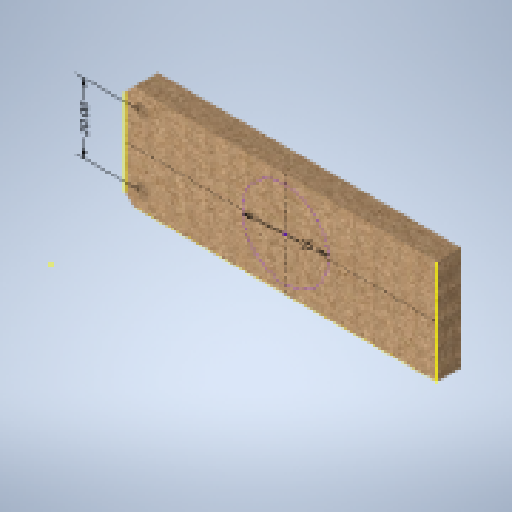
# Autodesk Inventor part: Dedo
Saved by Autodesk Inventor 2023.1 (Build 271208000, 208)
## iProperties
Created: 2022-10-28
Part Number: Dedo
Material: MDF Medium Density Fiberboard
Document SubType Name: Modeling
Designer: Daniel Peña
Density: 0.8 g/cm^3
Appearance: Cardboard - Corrugated
Author: Daniel Peña
Autodesk Inventor part; units mm, degrees
ref_plane "YZ Plane" through (0, 0, 0) normal (1, 0, 0) x (0, 1, 0)
ref_plane "XZ Plane" through (0, 0, 0) normal (0, 1, 0) x (-1, 0, 0)
ref_plane "XY Plane" through (0, 0, 0) normal (0, 0, 1) x (1, 0, 0)
sketch "Sketch1" plane through (0, 0, 0) normal (0, 0, 1) x (1, 0, 0)
  line L0 (23.8989, 56.2562) -> (111.3989, 56.2562)
  line L1 (111.3989, 56.2562) -> (111.3989, 26.2562)
  line L2 (111.3989, 26.2562) -> (23.8989, 26.2562)
  line L3 (21.3989, 28.7562) -> (21.3989, 53.7562)
  line L4 (21.3989, 53.7562) -> (23.8989, 56.2562)
  line L5 (21.3989, 28.7562) -> (23.8989, 26.2562)
  point P0 (0, 0)
  point P1 (21.3989, 56.2562)
  point P2 (21.3989, 26.2562)
  dimension "d0" = 30
  dimension "d1" = 90
  dimension "d2" = 2.5
  dimension "d3" = 2.5
  dimension "d4" = 2.5
  dimension "d5" = 2.5
  constraints: 12 end point, 4 point on line, 2 parallel, 1 horizontal, 1 perpendicular
  measures "d0" distance of L0.end L1.end
  measures "d1" distance of L1.end point (21.399, 26.256)
  measures "d2" distance of L3.end point (21.399, 56.256)
  measures "d3" distance of L0.start point (21.399, 56.256)
  measures "d4" distance of L3.start point (21.399, 26.256)
  measures "d5" distance of L2.end point (21.399, 26.256)
extrude "Extrusion1" add sketch "Sketch1" along normal blind 7
sketch "Sketch2" plane through (0, 0, 7) normal (0, 0, 1) x (1, 0, 0)
  line L0 (111.3989, 26.2562) -> (111.3989, 56.2562) construction
  line L1 (111.3989, 41.2562) -> (21.3989, 41.2562) construction
  line L2 (21.3989, 53.7562) -> (21.3989, 28.7562) construction
  line L3 (23.8989, 26.2562) -> (111.3989, 26.2562) projected
  point P0 (0, 0)
  point P1 (26.3989, 31.2562)
  point P2 (26.3989, 51.2562)
  dimension "d8" = 5
  dimension "d9" = 5
  constraints: 2 end point, 2 midpoint, 1 symmetric about line
  measures "d8" distance from line of L3 point (26.399, 31.256)
  measures "d9" distance from line of L2 point (26.399, 51.256)
hole "Hole1" at (26.3989, 31.2562, 7) at (26.3989, 51.2562, 7) direction (0, 0, -1) diameter 4 end through all
sketch "Sketch3" plane through (0, 0, 7) normal (0, 0, 1) x (1, 0, 0)
  circle A0 centre (67.6489, 41.2562) radius 12.5 construction
  line L0 (21.3989, 53.7562) -> (21.3989, 28.7562) projected
  line L1 (21.3989, 41.2562) -> (111.3989, 41.2562) construction
  line L2 (111.3989, 26.2562) -> (111.3989, 56.2562) projected
  line L3 (23.8989, 26.2562) -> (111.3989, 26.2562) construction
  line L4 (67.6489, 26.2562) -> (67.6489, 56.2562) construction
  point P0 (0, 0)
  dimension "d17" = 25
  constraints: 4 end point, 4 midpoint, 1 centre point, 1 coincident, 1 perpendicular
  measures "d17" diameter of A0
equation "\"d3\" = d2"
equation "\"d4\" = d2"
equation "\"d5\" = d4"
body "Solid1"
